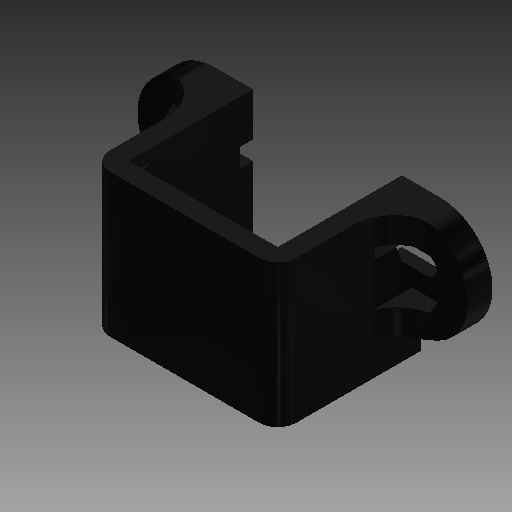
# Autodesk Inventor part: Mounting_bracket
Saved by Autodesk Inventor 2017 (Build 210142000, 142)
## iProperties
Created: 2011-05-27
Part Number: Mounting_bracket
Document SubType Name: Modeling
Designer: Hudy
Density: 1.06 g/cm^3
Material: ABS Plastic
Mass: 0.788054 g
Surface Area: 11.662 cm^2
Volume: 0.743447 cm^3
Appearance: Glossy - Black
Author: Hudy
Autodesk Inventor part; units mm, degrees
ref_plane "YZ Plane" through (0, 0, 0) normal (1, 0, 0) x (0, 1, 0)
ref_plane "XZ Plane" through (0, 0, 0) normal (0, 1, 0) x (-1, 0, 0)
sketch "Szkic1" plane through (0, 0, 0) normal (0, 0, 1) x (1, 0, 0)
  line L0 (-7.5, 5.75) -> (7.5, 5.75)
  line L1 (7.5, 5.75) -> (7.5, -5.75)
  line L2 (7.5, -5.75) -> (-7.5, -5.75)
  line L3 (-7.5, -5.75) -> (-7.5, 5.75)
  point P0 (0, 0)
  point P1 (0, 5.75)
  point P2 (-7.5, 0)
  dimension "d0" = 15
  dimension "d1" = 11.5
  constraints: 8 end point, 2 midpoint, 2 parallel, 1 horizontal, 1 horizontal alignment, 1 perpendicular, 1 vertical alignment
  measures "d0" distance of L1.end L2.end
  measures "d1" distance of L0.end L1.end
extrude "Wyciągnięcie proste1" add sketch "Szkic1" along normal blind 11.5
sketch "Szkic2" plane through (0, 0, 0) normal (0, 0, -1) x (-1, 0, 0)
  line L0 (7.5, 5.75) -> (-7.5, 5.75) projected
  line L1 (-7.5, 5.75) -> (-7.5, -5.75) projected
  line L2 (7.5, -5.75) -> (7.5, 5.75) projected
  line L3 (-13.3, 5.75) -> (13.3, 5.75)
  line L4 (13.3, 5.75) -> (13.3, -2.75)
  line L5 (13.3, -2.75) -> (-13.3, -2.75)
  line L6 (-13.3, -2.75) -> (-13.3, 5.75)
  point P0 (0, 0)
  dimension "d4" = 8.5
  dimension "d5" = 5.8
  dimension "d6" = 5.8
  constraints: 8 end point, 2 parallel, 1 collinear, 1 horizontal, 1 perpendicular
  measures "d4" distance of L5.end L3.start
  measures "d5" distance between parallel lines of L6 L1
  measures "d6" distance between parallel lines of L4 L2
extrude "Wyciągnięcie proste2" add sketch "Szkic2" against normal blind 2
fillet "Zaokrąglenie1" radius 4.25 4 edges at (-13.3, -2.75, 1) (-13.3, 5.75, 1) (13.3, -2.75, 1) (13.3, 5.75, 1)
fillet "Zaokrąglenie2" radius 1.5 2 edges at (-7.5, 0, 11.5) (7.5, 0, 11.5)
fillet "Zaokrąglenie3" radius 3.5 2 edges at (-7.5, 1.5, 2) (7.5, 1.5, 2)
ref_plane "Płaszczyzna konstrukcyjna1" through (0, 0, 1) normal (0, 0, -1) x (-1, 0, 0)
sketch "Szkic3" plane through (0, 0, 1) normal (0, 0, -1) x (-1, 0, 0)
  arc A0 (-9.05, 5.75) -> (-9.05, -2.75) centre (-9.05, 1.5) ccw projected
  arc A1 (9.05, -2.75) -> (9.05, 5.75) centre (9.05, 1.5) ccw projected
  line L0 (-6.55, 1.5) -> (-7.8, -0.6651)
  line L1 (-7.8, -0.6651) -> (-10.3, -0.6651)
  line L2 (-10.3, -0.6651) -> (-11.55, 1.5)
  line L3 (-11.55, 1.5) -> (-10.3, 3.6651)
  line L4 (-10.3, 3.6651) -> (-7.8, 3.6651)
  line L5 (-7.8, 3.6651) -> (-6.55, 1.5)
  line L6 (6.55, 1.5) -> (7.8, 3.6651)
  line L7 (7.8, 3.6651) -> (10.3, 3.6651)
  line L8 (10.3, 3.6651) -> (11.55, 1.5)
  line L9 (11.55, 1.5) -> (10.3, -0.6651)
  line L10 (10.3, -0.6651) -> (7.8, -0.6651)
  line L11 (7.8, -0.6651) -> (6.55, 1.5)
  point P0 (0, 0)
  dimension "d13" = 2.5
  dimension "d14" = 18.1
  constraints: 24 end point, 2 coincident, 1 equal length, 26 other
  measures "d13" distance of L3.end L4.end
  measures "d14" distance of A0.centre A1.centre
extrude "Wyciągnięcie proste3" cut sketch "Szkic3" against normal blind 3
sketch "Szkic4" plane through (0, 0, 0) normal (0, 0, -1) x (-1, 0, 0)
  arc A0 (-9.05, 5.75) -> (-9.05, -2.75) centre (-9.05, 1.5) ccw projected
  arc A1 (9.05, -2.75) -> (9.05, 5.75) centre (9.05, 1.5) ccw projected
  circle A2 centre (-9.05, 1.5) radius 0.75
  circle A3 centre (9.05, 1.5) radius 0.75
  line L0 (-9.05, 2.25) -> (9.05, 2.25)
  line L1 (9.05, 0.75) -> (-9.05, 0.75)
  point P0 (0, 0)
  dimension "d17" = 1.5
  constraints: 4 end point, 4 point on circle, 3 tangent, 2 centre point, 2 coincident, 1 equal radius
  measures "d17" diameter of A2
extrude "Wyciągnięcie proste4" cut sketch "Szkic4" against normal blind 1
sketch "Szkic5" plane through (0, 0, 0) normal (0, 0, -1) x (-1, 0, 0)
  line L0 (-7.5, -5.75) -> (7.5, -5.75) projected
  line L1 (9.05, 5.75) -> (-9.05, 5.75) projected
  line L2 (-6, -5.75) -> (6, -5.75)
  line L3 (6, -5.75) -> (6, 5.75)
  line L4 (6, 5.75) -> (-6, 5.75)
  line L5 (-6, 5.75) -> (-6, -5.75)
  point P0 (0, 0)
  point P1 (0, 5.75)
  dimension "d20" = 12
  constraints: 8 end point, 2 parallel, 2 point on line, 1 horizontal, 1 midpoint, 1 perpendicular, 1 vertical alignment
  measures "d20" distance of L3.end L4.end
extrude "Wyciągnięcie proste5" cut sketch "Szkic5" against normal blind 10
fillet "Zaokrąglenie4" radius 2 2 edges at (6, 0, 10) (-6, 0, 10)
sketch "Szkic7" plane through (0, 0, 0) normal (0, 0, -1) x (-1, 0, 0)
  line L0 (6, 5.75) -> (6, 2.25) projected
  line L1 (6, 0.75) -> (6, -5.75) projected
  line L2 (-6, 0.75) -> (-6, 2.25) projected
  line L3 (-6, 2.25) -> (-6, 5.75) projected
  line L4 (-6, -5.75) -> (-6, 0.75) projected
  line L5 (6, 2.25) -> (6, 0.75) projected
  line L6 (-6, 5.75) -> (6, 5.75)
  line L7 (6, 5.75) -> (6, 4.75)
  line L8 (6, 4.75) -> (-6, 4.75)
  line L9 (-6, 4.75) -> (-6, 5.75)
  line L10 (-6, 0.75) -> (6, 0.75)
  line L11 (6, 0.75) -> (6, -0.25)
  line L12 (6, -0.25) -> (-6, -0.25)
  line L13 (-6, -0.25) -> (-6, 0.75)
  line L14 (-6, -5.75) -> (6, -5.75)
  line L15 (6, -5.75) -> (6, -2.25)
  line L16 (6, -2.25) -> (-6, -2.25)
  line L17 (-6, -2.25) -> (-6, -5.75)
  point P0 (0, 0)
  dimension "d29" = 1
  dimension "d30" = 1
  dimension "d31" = 4
  dimension "d32" = 2
  constraints: 24 end point, 6 parallel, 4 point on line, 3 horizontal, 3 perpendicular
  measures "d29" distance of L6.end L7.end
  measures "d30" distance of L10.end L11.end
  measures "d31" distance between parallel lines of L8 L10
  measures "d32" distance between parallel lines of L16 L12
extrude "Wyciągnięcie proste7" cut sketch "Szkic7" against normal blind 10 contours L0 L8 L3 L6 | L1 L12 L4 L10 | L1 L14 L4 L16
equation "\"d6\" = d5"
